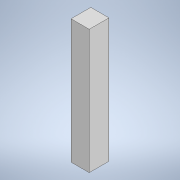
# Autodesk Inventor part: Cloth
Saved by Autodesk Inventor 2020 (Build 240168000, 168)
## iProperties
Created: 2021-07-16
Part Number: Cloth
Material: Generic
Document SubType Name: Modeling
Designer: pc
Density: 1 g/cm^3
Appearance: Default
Author: pc
Autodesk Inventor part; units mm, degrees
ref_plane "YZ Plane" through (0, 0, 0) normal (1, 0, 0) x (0, 1, 0)
ref_plane "XZ Plane" through (0, 0, 0) normal (0, 1, 0) x (-1, 0, 0)
ref_plane "XY Plane" through (0, 0, 0) normal (0, 0, 1) x (1, 0, 0)
sketch "Sketch1" plane through (0, 0, 0) normal (1, 0, 0) x (0, 1, 0)
  line L0 (10.5872, 8.0541) -> (-388.1928, 8.0541)
  line L1 (-388.1928, 8.0541) -> (-388.1928, -55.4459)
  line L2 (-388.1928, -55.4459) -> (10.5872, -55.4459)
  line L3 (10.5872, -55.4459) -> (10.5872, 8.0541)
  point P0 (0, 0)
  dimension "d0" = 398.78
  dimension "d1" = 63.5
  constraints: 8 end point, 2 parallel, 1 horizontal, 1 perpendicular
  measures "d0" distance of L2.end L1.end
  measures "d1" distance of L1.end L0.end
extrude "Extrusion1" add sketch "Sketch1" along normal blind 58.42
body "Solid1"
